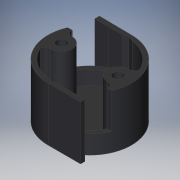
# Autodesk Inventor part: BatteryIsolator
Saved by Autodesk Inventor 2017 SP1 (Build 210196100, 196)
## iProperties
Created: 2021-08-14
Part Number: BatteryIsolator
Material: Generic
Document SubType Name: Modeling
Designer: togenshi
Density: 1 g/cm^3
Appearance: Default
Author: togenshi
Autodesk Inventor part; units mm, degrees
ref_plane "YZ Plane" through (0, 0, 0) normal (1, 0, 0) x (0, 1, 0)
ref_plane "XZ Plane" through (0, 0, 0) normal (0, 1, 0) x (-1, 0, 0)
ref_plane "XY Plane" through (0, 0, 0) normal (0, 0, 1) x (1, 0, 0)
sketch "Sketch1" plane through (0, 0, 0) normal (0, 0, 1) x (1, 0, 0)
  circle A0 centre (0, 0) radius 29.5
  circle A1 centre (20, 0) radius 3.375
  circle A2 centre (-20, 0) radius 3.375
  line L0 (0, -27.5) -> (-4.0078, -26.1952)
  line L1 (0, -27.5) -> (4.0078, -26.1952)
  arc A3 (-24.1091, -11) -> (-4.0078, -26.1952) centre (0, 0) ccw
  arc A4 (4.0078, -26.1952) -> (24.1091, -11) centre (0, 0) ccw
  line L2 (4.0076, 26.1952) -> (0, 27.5)
  line L3 (0, 27.5) -> (-4.0076, 26.1952)
  arc A5 (24.1091, 11) -> (4.0076, 26.1952) centre (0, 0) ccw
  arc A6 (-4.0076, 26.1952) -> (-24.1091, 11) centre (0, 0) ccw
  arc A7 (20.1829, 7.4978) -> (20.1829, -7.4978) centre (20, 0) ccw
  arc A8 (-20.1829, -7.4978) -> (-20.1829, 7.4978) centre (-20, 0) ccw
  arc A9 (-20, -7.5) -> (-24.1091, -11) centre (-20.1402, -11.4975) ccw
  arc A10 (-24.1091, 11) -> (-20, 7.5) centre (-20.1402, 11.4975) ccw
  arc A11 (24.1091, -11) -> (20, -7.5) centre (20.1402, -11.4975) ccw
  arc A12 (20, 7.5) -> (24.1091, 11) centre (20.1402, 11.4975) ccw
  dimension "d46" = 59
  dimension "d49" = 6.75
  dimension "d50" = 6.75
  dimension "d105" = 4
  dimension "d106" = 4
  dimension "d107" = 4
  dimension "d109" = 4
  constraints: 28 point on circle, 13 centre point, 8 end point, 1 coincident
  measures "d46" diameter of A0
  measures "d49" diameter of A1
  measures "d50" diameter of A2
  measures "d105" radius of A9
  measures "d106" radius of A10
  measures "d107" radius of A11
  measures "d109" radius of A12
extrude "Extrusion1" add sketch "Sketch1" along normal blind 35
sketch "Sketch9" plane through (0, 0, 0) normal (0, 0, -1) x (-1, 0, 0)
  circle A0 centre (-20, 0) radius 3.375
  circle A1 centre (20, 0) radius 3.375
  line L0 (20, -6.5) -> (25.6292, -3.25)
  line L1 (25.6292, -3.25) -> (25.6292, 3.25)
  line L2 (25.6292, 3.25) -> (20, 6.5)
  line L3 (20, 6.5) -> (14.3708, 3.25)
  line L4 (14.3708, 3.25) -> (14.3708, -3.25)
  line L5 (14.3708, -3.25) -> (20, -6.5)
  line L6 (-20, -6.5) -> (-14.3708, -3.25)
  line L7 (-14.3708, -3.25) -> (-14.3708, 3.25)
  line L8 (-14.3708, 3.25) -> (-20, 6.5)
  line L9 (-20, 6.5) -> (-25.6292, 3.25)
  line L10 (-25.6292, 3.25) -> (-25.6292, -3.25)
  line L11 (-25.6292, -3.25) -> (-20, -6.5)
  point P0 (0, 0)
  point P1 (0, 0)
  constraints: 24 end point, 6 parallel, 2 centre point, 2 coincident, 2 vertical
extrude "Extrusion11" cut sketch "Sketch9" against normal blind 3
extrude "Extrusion12" add sketch "Sketch1" against normal blind 3 contours A0 | L0 A3 A9 A8 A10 A6 L3 L2 A5 A12 A7 A11 A4 L1
extrude "Extrusion13" cut sketch "Sketch9" along normal blind 3
sketch "Sketch10" plane through (0, 0, 35) normal (0, 0, 1) x (1, 0, 0)
  arc A0 (-24.1091, -11) -> (-4.0078, -26.1952) centre (0, 0) ccw projected
  line L0 (0, -26.5) -> (12.9615, -26.5)
  line L1 (27.1662, -11.5) -> (23.8747, -11.5)
  arc A1 (24.1091, 11) -> (4.0076, 26.1952) centre (0, 0) ccw projected
  line L2 (0, 26.5) -> (-12.9615, 26.5)
  line L3 (-27.1662, 11.5) -> (-23.8747, 11.5)
  arc A2 (12.9615, -26.5) -> (27.1662, -11.5) centre (0, 0) ccw
  arc A3 (-12.9615, 26.5) -> (-27.1662, 11.5) centre (0, 0) ccw
  arc A4 (0, -26.5) -> (23.8747, -11.5) centre (0, 0) ccw
  arc A5 (0, 26.5) -> (-23.8747, 11.5) centre (0, 0) ccw
  point P0 (24.1091, -11)
  point P1 (-24.1091, 11)
  constraints: 10 point on circle, 8 end point, 4 centre point, 3 tangent, 2 coincident, 2 horizontal
extrude "Extrusion14" cut sketch "Sketch10" against normal blind 25
sketch "Sketch11" plane through (0, 0, 35) normal (0, 0, 1) x (1, 0, 0)
  line L0 (12.9615, -26.5) -> (3.0715, -26.5) projected
  line L1 (12.9615, -26.5) -> (22.9615, -26.5)
  line L2 (22.9615, -26.5) -> (22.9615, -29.5)
  arc A0 (-27.1662, 11.5) -> (12.9615, -26.5) centre (0, 0) ccw projected
  line L3 (0, -29.5) -> (22.9615, -29.5)
  line L4 (12.9615, -26.5) -> (3.0715, -26.5)
  line L5 (3.0715, -26.5) -> (0, -27.5) projected
  line L6 (0, -27.5) -> (0, -29.5)
  circle A1 centre (0, 0) radius 29.5 projected
  line L7 (-12.9667, 26.4974) -> (-22.9667, 26.4974)
  line L8 (-22.9667, 26.4974) -> (-22.9667, 29.7944)
  line L9 (0, 29.5) -> (-22.9667, 29.7944)
  line L10 (-12.9667, 26.4974) -> (-3.0793, 26.4974)
  line L11 (0, 27.5) -> (-4.0076, 26.1952) projected
  line L12 (0, 27.5) -> (0, 29.5)
  dimension "d93" = 10
  dimension "d94" = 10
  constraints: 20 end point, 4 horizontal, 4 perpendicular, 3 point on circle, 2 point on line, 1 tangent
  measures "d93" distance of L0.start L1.end
  measures "d94" distance of L7.start L7.end
extrude "Extrusion15" add sketch "Sketch11" against normal blind 38 contours A0 L6 L5 L0 | L1 L2 L3 A0 | A1 L7 L8 L9
body "Solid1"
